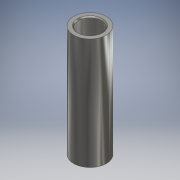
# Autodesk Inventor part: TULEJKA
Saved by Autodesk Inventor 2017 SP1 (Build 210196100, 196)
## iProperties
Created: 2021-02-07
Part Number: TULEJKA
Material: Stal nierdzewna
Document SubType Name: Modeling
Designer: Napoleon
Mass: 4.48041 g
Surface Area: 10.3728 cm^2
Volume: 0.560051 cm^3
Density: 8 g/cm^3
Appearance: Częściowo polerowany
Author: Napoleon
Autodesk Inventor part; units mm, degrees
ref_plane "YZ Plane" through (0, 0, 0) normal (1, 0, 0) x (0, 1, 0)
ref_plane "XZ Plane" through (0, 0, 0) normal (0, 1, 0) x (-1, 0, 0)
ref_plane "XY Plane" through (0, 0, 0) normal (0, 0, 1) x (1, 0, 0)
sketch "Szkic1" plane through (0, 0, 0) normal (0, 0, 1) x (1, 0, 0)
  circle A0 centre (0, 0) radius 3.7
  circle A1 centre (0, 0) radius 2.575
  dimension "d0" = 7.4
  dimension "d1" = 5.15
  constraints: 2 centre point, 2 coincident
  measures "d0" diameter of A0
  measures "d1" diameter of A1
extrude "Wyciągnięcie proste1" add sketch "Szkic1" along normal mid plane 25.3
chamfer "Faza1" distance 0.25 angle 45 2 edges at (-2.575, 0, 12.65) (-2.575, 0, -12.65)
